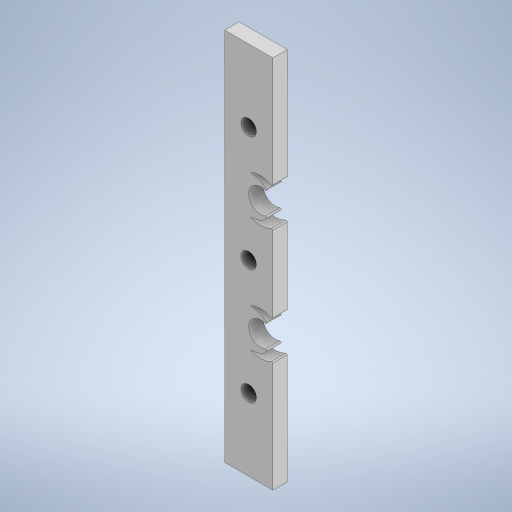
# Autodesk Inventor part: cover_setter_side_front
Saved by Autodesk Inventor 2024.1 (Build 281209000, 209)
## iProperties
Created: 2025-03-07
Part Number: cover_setter_side_front
Material: 一般
Document SubType Name: Modeling
Designer: hibik
Density: 1 g/cm^3
Appearance: 既定
Author: hibik
Autodesk Inventor part; units mm, degrees
ref_plane "YZ Plane" through (0, 0, 0) normal (1, 0, 0) x (0, 1, 0)
ref_plane "XZ Plane" through (0, 0, 0) normal (0, 1, 0) x (-1, 0, 0)
ref_plane "XY Plane" through (0, 0, 0) normal (0, 0, 1) x (1, 0, 0)
sketch "スケッチ1" plane through (0, 0, 0) normal (0, 0, 1) x (1, 0, 0)
  line L0 (-5, 39) -> (5, 39)
  line L1 (5, 39) -> (5, -39)
  line L2 (5, -39) -> (-5, -39)
  line L3 (-5, -39) -> (-5, 39)
  circle A0 centre (0, 24) radius 1.6
  circle A1 centre (0, 0) radius 1.6
  circle A2 centre (0, -24) radius 1.6
  dimension "d0" = 3.2
  dimension "d1" = 15
  dimension "d2" = 24
  dimension "d3" = 24
  dimension "d4" = 5
  dimension "d5" = 15
  dimension "d6" = 10
  constraints: 8 end point, 3 centre point, 2 equal radius, 2 parallel, 2 vertical alignment, 1 coincident, 1 horizontal, 1 perpendicular
  measures "d0" diameter of A0
  measures "d1" distance from line of L0 A0.centre
  measures "d2" distance of A1.centre A0.centre
  measures "d3" distance of A2.centre A1.centre
  measures "d4" distance from line of L1 A0.centre
  measures "d5" distance from line of L2 A2.centre
  measures "d6" distance of L0.start L0.end
extrude "押し出し1" add sketch "スケッチ1" along normal blind 3
sketch "スケッチ2" plane through (0, 0, 3) normal (0, 0, 1) x (1, 0, 0)
  circle A0 centre (2.5, 12) radius 2.5
  line L0 (2.5, 12) -> (5, 14.5)
  line L1 (2.5, 12) -> (5, 9.5)
  line L2 (2.5, 12) -> (5, 12)
  line L3 (5, -39) -> (5, 39) projected
  circle A1 centre (0, 24) radius 1.6 projected
  circle A2 centre (0.6796, 12) radius 4
  circle A3 centre (2.5, 12) radius 4.5
  point P0 (0, 0)
  point P1 (4.2678, 13.7678)
  point P2 (4.2678, 10.2322)
  point P3 (0.4225, 8.0083)
  point P4 (5, 8.2583)
  point P5 (5, 15.7417)
  point P6 (0.4225, 15.9917)
  dimension "d9" = 5
  dimension "d12" = 8
  dimension "d10" = 45
  dimension "d11" = 12
  dimension "d13" = 9
  constraints: 6 end point, 4 point on line, 1 centre point, 1 coincident, 1 horizontal, 1 horizontal alignment, 1 perpendicular, 1 vertical, 6 other
  measures "d10" angle of L2 L0
  measures "d11" vertical distance of A1.centre L0.start
  measures "d13" diameter of A3
extrude "押し出し2" cut sketch "スケッチ2" against normal through all contours L2 A2 A0 | L3 L1 A0 | A0 A2 L2 | A0 L0 L3 | L0 L1 A0 | A2 L2 L0 | A2 A3 L3 L0 | L1 L3 A3 A2 | L1 L2 A2
fillet "フィレット1" radius 0.2 4 edges at (4.2678, 13.7678, 1.5) (4.2678, 10.2322, 1.5) (5, 15.7417, 1.5) (5, 8.2583, 1.5)
mirror "ミラー1" about plane through (0, 0, 0) normal (0, 1, 0) of "押し出し2", "フィレット1"
